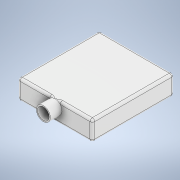
# Autodesk Inventor part: WaterContainer
Saved by Autodesk Inventor 2020 (Build 240168000, 168)
## iProperties
Created: 2020-04-09
Part Number: WaterContainer
Material: Типовые
Document SubType Name: Modeling
Designer: Михаил
Density: 1 g/cm^3
Appearance: По умолчанию
Author: Михаил
Autodesk Inventor part; units mm, degrees
ref_plane "YZ Plane" through (0, 0, 0) normal (1, 0, 0) x (0, 1, 0)
ref_plane "XZ Plane" through (0, 0, 0) normal (0, 1, 0) x (-1, 0, 0)
ref_plane "XY Plane" through (0, 0, 0) normal (0, 0, 1) x (1, 0, 0)
sketch "Эскиз1" plane through (0, 0, 0) normal (0, 1, 0) x (-1, 0, 0)
  line L0 (0, 0) -> (320, 0)
  line L1 (320, 0) -> (320, -350)
  line L2 (320, -350) -> (0, -350)
  line L3 (0, -350) -> (0, 0)
  dimension "d0" = 320
  dimension "d1" = 350
  constraints: 8 end point, 2 parallel, 1 horizontal, 1 perpendicular
  measures "d0" distance of L1.end L2.end
  measures "d1" distance of L0.end L1.end
extrude "Выдавливание1" add sketch "Эскиз1" along normal blind 85
sketch "Эскиз3" plane through (-320, 0, 0) normal (0, 0, 1) x (1, 0, 0)
  circle A0 centre (160, 55) radius 30
  line L0 (0, 0) -> (320, 0) projected
  dimension "d7" = 60
  dimension "d8" = 160
  dimension "d9" = 55
  constraints: 1 centre point
  measures "d7" diameter of A0
  measures "d8" horizontal distance of L0.end A0.centre
  measures "d9" distance from line of L0 A0.centre
extrude "Выдавливание2" add sketch "Эскиз3" along normal blind 50
fillet "Сопряжение1" radius 10 13 edges at (0, 85, -175) (-80, 85, 0) (-240, 85, 0) (0, 42.5, 0) (0, 0, -175) (0, 42.5, -350) (-160, 85, -350) (-160, 0, 0) (-320, 85, -175) (-320, 42.5, 0) (-320, 0, -175) (-320, 42.5, -350) (-160, 0, -350)
sketch "Эскиз4" plane through (-160, 55, 50) normal (0, 0, 1) x (1, 0, 0)
  circle A0 centre (0, 0) radius 25
  point P0 (160, -55)
  dimension "d13" = 50
  constraints: 1 centre point
  measures "d13" diameter of A0
extrude "Выдавливание3" cut sketch "Эскиз4" against normal blind 50
